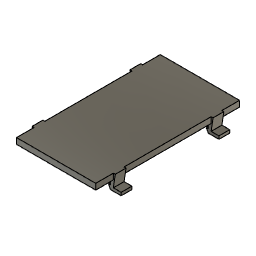
couvercle_cage_controlleur v6 (Autodesk Fusion 360 design; units mm, degrees)
Autodesk Fusion 360 part; units mm, degrees
sketch "Esquisse1" plane through (0, 0, 0) normal (0, 0, 1) x (1, 0, 0)
  line L0 (-11.8169, 52.5158) -> (25.6831, 52.5158)
  line L1 (-9.8169, -15.8592) -> (-9.8169, 50.6408)
  line L2 (-11.8169, -17.9842) -> (-11.8169, 52.5158)
  line L3 (23.6831, -15.8592) -> (-9.8169, -15.8592)
  line L4 (23.6831, 50.6408) -> (23.6831, -15.8592)
  line L5 (-9.8169, 50.6408) -> (23.6831, 50.6408)
  line L6 (25.6831, 52.5158) -> (25.6831, -17.9842)
  line L7 (25.6831, -17.9842) -> (-11.8169, -17.9842)
  line L8 (-13.3169, 54.0158) -> (27.1831, 54.0158)
  line L9 (27.1831, 54.0158) -> (27.1831, -19.4842)
  line L10 (27.1831, -19.4842) -> (-13.3169, -19.4842)
  line L11 (-13.3169, -19.4842) -> (-13.3169, 54.0158)
  line L12 (25.4331, 52.2658) -> (25.4331, -17.7342) construction
  line L13 (-11.5669, -17.7342) -> (-11.5669, 52.2658) construction
  line L14 (-11.5669, 52.2658) -> (25.4331, 52.2658) construction
  line L15 (25.4331, -17.7342) -> (-11.5669, -17.7342) construction
  line L16 (-11.5669, 17.2658) -> (25.4331, 17.2658) construction
  line L17 (4.1831, -17.9842) -> (9.6831, -17.9842)
  line L18 (-13.3169, -19.4842) -> (27.1831, -19.4842)
  line L19 (25.4331, 46.2658) -> (24.4331, 46.2658) construction
  line L20 (24.4331, 46.2658) -> (24.4331, 38.2658) construction
  line L21 (24.4331, 38.2658) -> (25.4331, 38.2658) construction
  line L22 (25.4331, 38.2658) -> (25.4331, 46.2658) construction
  line L23 (6.9331, 17.2658) -> (6.9331, 52.2658) construction
  line L24 (-11.5669, 46.2658) -> (-10.5669, 46.2658) construction
  line L25 (-10.5669, 46.2658) -> (-10.5669, 38.2658) construction
  line L26 (-10.5669, 38.2658) -> (-11.5669, 38.2658) construction
  line L27 (-11.5669, -11.7342) -> (-10.5669, -11.7342) construction
  line L28 (-10.5669, -11.7342) -> (-10.5669, -3.7342) construction
  line L29 (-10.5669, -3.7342) -> (-11.5669, -3.7342) construction
  line L30 (24.4331, -11.7342) -> (24.4331, -3.7342) construction
  line L31 (25.4331, -11.7342) -> (24.4331, -11.7342) construction
  line L32 (24.4331, -3.7342) -> (25.4331, -3.7342) construction
  line L33 (31.1831, 45.0158) -> (24.6831, 45.0158)
  line L34 (24.6831, 45.0158) -> (24.6831, 39.5158)
  line L35 (24.6831, 39.5158) -> (31.1831, 39.5158)
  line L36 (31.1831, 39.5158) -> (31.1831, 45.0158)
  line L37 (-17.3169, 39.5158) -> (-17.3169, 45.0158)
  line L38 (-17.3169, 45.0158) -> (-10.8169, 45.0158)
  line L39 (-10.8169, 45.0158) -> (-10.8169, 39.5158)
  line L40 (-10.8169, 39.5158) -> (-17.3169, 39.5158)
  line L41 (24.6831, -10.4842) -> (24.6831, -4.9842)
  line L42 (31.1831, -10.4842) -> (24.6831, -10.4842)
  line L43 (31.1831, -4.9842) -> (31.1831, -10.4842)
  line L44 (24.6831, -4.9842) -> (31.1831, -4.9842)
  line L45 (-10.8169, -4.9842) -> (-17.3169, -4.9842)
  line L46 (-17.3169, -4.9842) -> (-17.3169, -10.4842)
  line L47 (-17.3169, -10.4842) -> (-10.8169, -10.4842)
  line L48 (-10.8169, -10.4842) -> (-10.8169, -4.9842)
  point P0 (76.3509, -9.9514)
  dimension "d1" = 33.5
  dimension "d2" = 66.5
  dimension "d3" = 70.5
  dimension "d4" = 37.5
  dimension "d7" = 1.5
  dimension "d8" = 1.5
  dimension "d9" = 1.5
  dimension "d15" = 2
  dimension "d16" = 1.875
  dimension "d19" = 70
  dimension "d20" = 37
  dimension "d24" = 0.25
  dimension "d25" = 0.25
  dimension "d59" = 1
  dimension "d60" = 8
  dimension "d61" = 21
  dimension "d81" = 4
  dimension "d82" = 1
  dimension "d83" = 5.5
  dimension "d84" = 1.25
  constraint horizontal L5
  constraint vertical L4
  constraint horizontal L3
  constraint vertical L1
  constraint horizontal L0
  constraint vertical L6
  constraint horizontal L7
  constraint vertical L2
  constraint horizontal L8
  constraint vertical L9
  constraint horizontal L10
  constraint vertical L11
  constraint horizontal L14
  constraint vertical L12
  constraint horizontal L15
  constraint vertical L13
  constraint midpoint L13 L16.start
  constraint midpoint L12 L16.end
  constraint symmetric L8.start L16 L10.end
  constraint symmetric L8.end L16 L9.end
  constraint horizontal L19
  constraint vertical L20
  constraint horizontal L21
  constraint vertical L22
  constraint coincident L12 L19.start
  constraint midpoint L16 L23.start
  constraint midpoint L14 L23.end
  constraint symmetric L19.start L23 L24.start
  constraint symmetric L19.end L23 L24.end
  constraint symmetric L20.end L23 L25.end
  constraint symmetric L21.end L23 L26.end
  constraint symmetric L16 L19.start L31.start
  constraint symmetric L16 L19.end L30.start
  constraint symmetric L16 L20.end L30.end
  constraint symmetric L16 L21.end L32.end
  constraint symmetric L16 L24.start L27.start
  constraint symmetric L16 L24.end L27.end
  constraint symmetric L16 L25.end L28.end
  constraint symmetric L16 L26.end L29.end
  constraint horizontal L33
  constraint vertical L34
  constraint horizontal L35
  constraint vertical L36
  constraint symmetric L23 L33.start L37.end
  constraint symmetric L23 L33.end L38.end
  constraint symmetric L23 L34.end L39.end
  constraint symmetric L23 L35.end L37.start
  constraint symmetric L16 L33.start L42.start
  constraint symmetric L16 L33.end L41.start
  constraint symmetric L16 L34.end L41.end
  constraint symmetric L16 L35.end L43.start
  constraint symmetric L16 L37.start L45.end
  constraint symmetric L16 L37.end L46.end
  constraint symmetric L16 L38.end L47.end
  constraint symmetric L16 L39.end L45.start
  measures "d1" distance of L1 L4
  measures "d2" distance of L3 L5
  measures "d3" distance of L0 L7
  measures "d4" distance of L2 L6
  measures "d7" distance of L0 L8
  measures "d8" distance of L7 L10
  measures "d9" distance of L6 L9
  measures "d15" distance of L4 L6
  measures "d16" distance of L0 L5
  measures "d19" distance of L14 L15
  measures "d20" distance of L12 L13
  measures "d24" distance of L2 L13
  measures "d25" distance of L0 L14
  measures "d59" distance of L20 L22
  measures "d60" distance of L19 L21
  measures "d61" distance of L16 L21
  measures "d81" distance of L9 L36
  measures "d82" distance of L6 L34
  measures "d83" distance of L33 L35
  measures "d84" distance of L19 L33
extrude "Extrusion1" add sketch "Esquisse1" along normal blind 1 contours L0 L2 L6 L8 L9 L11 L33 L38 | L0 L2 L6 L7 L17 L33 L34 L35 L38 L39 L40 L41 L42 L44 L45 L47 L48 | L2 L38 L39 L40 | L2 L11 L38 L40 | L6 L9 L33 L35 | L6 L33 L34 L35 | L2 L11 L40 L45 | L6 L9 L35 L44 | L2 L45 L47 L48 | L2 L11 L45 L47 | L6 L9 L42 L44 | L6 L41 L42 L44 | L2 L6 L7 L9 L10 L11 L17 L18 L42 L47 | L1 L3 L4 L5 makes body 1
extrude "Extrusion2" add sketch "Esquisse1" against normal blind 2.5 contours L0 L2 L6 L8 L9 L11 L33 L38 | L2 L11 L38 L40 | L6 L9 L33 L35 | L2 L11 L40 L45 | L6 L9 L35 L44 | L2 L11 L45 L47 | L6 L9 L42 L44 | L2 L6 L7 L9 L10 L11 L17 L18 L42 L47 bodies 1
extrude "Extrusion3" add sketch "Esquisse1" against normal blind 5 from surface at -2 separate body contours L2 L11 L38 L40 | L6 L9 L33 L35 | L2 L11 L45 L47 | L6 L9 L42 L44 makes body 2 at (-11.8169, 41.3491, -3.6667) makes body 3 at (27.1831, 43.1825, -3.6667) makes body 4 at (-11.8169, -8.6509, -3.6667) makes body 5 at (27.1831, -6.8175, -5.3333)
extrude "Extrusion4" add sketch "Esquisse1" along normal blind 1.5 from surface at -7 contours L11 L37 L38 L40 | L9 L33 L35 L36 | L11 L45 L46 L47 | L9 L42 L43 L44 bodies 2 3 4 5
extrude "Extrusion5" add sketch "Esquisse1" against normal blind 2 from surface at -5 contours L2 L38 L39 L40 | L6 L33 L34 L35 | L2 L45 L47 L48 | L6 L41 L42 L44 bodies 2 3 4 5
extrude "Extrusion7" cut 1 faces at (-12.8169, 29.0158, -2.5) along direction (0, 0, 1) blind 0.5 on bodies 1 bodies 1
extrude "Extrusion9" add sketch "Esquisse1" against normal blind 1.5 separate body contours L1 L3 L4 L5 makes body 6
sketch "Esquisse6" plane through (0, -10.4842, 0) normal (0, -1, 0) x (1, 0, 0)
  line L0 (27.1831, -2) -> (25.6831, -2)
  line L1 (25.6831, -2) -> (25.6831, -5)
  line L2 (25.6831, -5) -> (24.6831, -5)
  line L3 (24.6831, -5) -> (24.6831, -7)
  line L4 (24.6831, -7) -> (31.1831, -7)
  line L5 (31.1831, -7) -> (31.1831, -5.5)
  line L6 (31.1831, -5.5) -> (27.1831, -5.5)
  line L7 (27.1831, -5.5) -> (27.1831, -2)
  line L8 (27.1831, -2) -> (-13.3169, -2) construction
  line L9 (-13.3169, -2) -> (-13.3169, -5.5)
  line L10 (6.9331, -2) -> (6.9331, -9) construction
  line L11 (27.1831, -5.5) -> (27.1831, 1)
  line L12 (27.1831, 1) -> (28.1831, 1)
  line L13 (28.1831, 1) -> (27.1831, -5.5)
  line L14 (25.6831, -7) -> (24.6831, -5)
  line L15 (24.6831, -5) -> (24.6831, -7)
  line L16 (24.6831, -7) -> (25.6831, -7)
  line L17 (-14.3169, 1) -> (-13.3169, -5.5)
  line L18 (-13.3169, -5.5) -> (-13.3169, 1)
  line L19 (-11.8169, -7) -> (-10.8169, -5)
  line L20 (-10.8169, -7) -> (-11.8169, -7)
  line L21 (-10.8169, -5) -> (-10.8169, -7)
  line L22 (-13.3169, 1) -> (-14.3169, 1)
  dimension "d85" = 1
  constraint coincident L0.start L7.end
  constraint perpendicular L1 L8
  constraint coincident L8.end L9
  constraint midpoint L8 L10.start
  constraint perpendicular L8 L10
  constraint coincident L6.end L7.start
  constraint perpendicular L6 L11
  constraint perpendicular L11 L12
  constraint coincident L4 L14.start
  constraint coincident L2.end L3.start
  constraint coincident L3.end L4.start
  constraint symmetric L10 L6.end L9.end
  constraint symmetric L10 L11.end L18.end
  constraint symmetric L10 L12.end L17.start
  constraint symmetric L10 L14.start L19.start
  constraint symmetric L10 L2.end L19.end
  constraint symmetric L10 L3.end L20.start
  measures "d85" distance of L11.end L12.end
extrude "Extrusion12" cut sketch "Esquisse6" against normal up to surface (55.5 mm away) contours L3 L4 L14 L15 L16 | L19 L20 L21 bodies 2 3 4 5
extrude "Extrusion13" add sketch "Esquisse6" against normal up to surface (5.5 mm away) contours L7 L11 L12 L13 | L9 L17 L18 L22 bodies 1 4 5
extrude "Extrusion14" add sketch "Esquisse6" against normal up to surface (5.5 mm away) from surface at -50 contours L7 L11 L12 L13 | L9 L17 L18 L22 bodies 1 2 3
